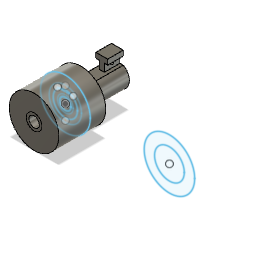
CoilWinder (Autodesk Fusion 360 design; units mm, degrees)
Autodesk Fusion 360 part; units mm, degrees
note: some values were not read from the file. Set by a fixed rule: which sketch regions a step uses.
sketch "Adapter_3mm" plane through (0, 0, 0) normal (0, 0, 1) x (1, 0, 0) in component "Deprecated - Adapter1"
  circle A0 centre (0, 0) radius 1
  circle A1 centre (0, 0) radius 1.5
  circle A2 centre (0, 0) radius 2.3
  circle A3 centre (0, 0) radius 4.7625
  dimension "d1" = 2
  dimension "d2" = 3
  dimension "d3" = 4.6
  dimension "d48" = 9.525
  constraint coincident A0.centre A1.centre
  constraint concentric A0 A1
  constraint concentric A1 A3
  measures "d1" diameter of A0
  measures "d2" diameter of A1
  measures "d3" diameter of A2
  measures "d48" diameter of A3
extrude "Extrude1" add sketch "Adapter_3mm" against normal blind 12 contours A1 | A2 makes body 1 in component "Deprecated - Adapter1"
extrude "Extrude2" add sketch "Adapter_3mm" along normal blind 7 contours A2 bodies 1 in component "Deprecated - Adapter1"
sketch "Face" plane through (0, 0, 0) normal (0, 0, 1) x (1, 0, 0) in component "StepperMount"
  line L0 (0, 0) -> (17.4625, 0) construction
  circle A0 centre (17.4625, 0) radius 1.8
  circle A1 centre (0, 0) radius 4.75
  line L1 (0, 0) -> (0, -15)
  line L2 (0, -15) -> (25, -15)
  line L3 (25, -15) -> (25, 10)
  line L4 (25, 10) -> (0, 10)
  line L5 (0, 10) -> (0, -15)
  line L6 (-25, 10) -> (0, 10)
  line L7 (-25, -15) -> (-25, 10)
  line L8 (0, -15) -> (-25, -15)
  circle A2 centre (-17.4625, 0) radius 1.8
  point P0 (-17.4625, 0)
  dimension "d8" = 17.4625
  dimension "d9" = 3.6
  dimension "d10" = 9.5
  dimension "d11" = 15
  dimension "d12" = 25
  dimension "d13" = 25
  constraint horizontal L0
  constraint coincident L0.start A1.centre
  constraint coincident L0.end A0.centre
  constraint perpendicular L0 L1
  constraint horizontal L2
  constraint vertical L3
  constraint horizontal L4
  constraint vertical L5
  constraint symmetric L0.end L5 P0
  constraint symmetric A0 L5 A2
  constraint symmetric L1.end L5 L2.start
  constraint symmetric L2.end L5 L7.start
  constraint symmetric L3.end L5 L6.start
  constraint symmetric L4.end L5 L6.end
  measures "d8" distance of L0.start L0.end
  measures "d9" diameter of A0
  measures "d10" diameter of A1
  measures "d11" distance of L0.start L1.end
  measures "d12" distance of L1.end L2.end
  measures "d13" distance of L1.end L4.end
ref_plane "WorkPlane1" through (0, -15, 0) normal (0, 1, 0) x (0, 0, 1) in component "StepperMount"
sketch "Base" plane through (0, -15, 0) normal (0, 1, 0) x (1, 0, 0) in component "StepperMount"
  line L0 (0, 0) -> (-25, 0)
  line L1 (0, 0) -> (25, 0)
  line L2 (0, 0) -> (25, 0)
  line L3 (25, 0) -> (25, 18)
  line L4 (25, 18) -> (0, 18)
  line L5 (0, 18) -> (0, 0)
  line L6 (0, 12.9238) -> (19, 12.9238) construction
  circle A0 centre (19, 12.9238) radius 0.95
  line L7 (25, 0) -> (23.4, 0)
  line L8 (23.4, 0) -> (23.4, 18)
  line L9 (23.4, 18) -> (25, 18)
  line L10 (25, 18) -> (25, 0)
  line L11 (-25, 18) -> (0, 18)
  circle A1 centre (-19, 12.9238) radius 0.95
  line L12 (-25, 0) -> (-25, 18)
  line L13 (-23.4, 0) -> (-23.4, 18)
  line L14 (-23.4, 18) -> (-25, 18)
  line L15 (25, 12) -> (30.7822, 8)
  point P0 (-19, 12.9238)
  dimension "d17" = 25
  dimension "d18" = 18
  dimension "d19" = 1.9
  dimension "d20" = 1.6
  dimension "d21" = 18
  constraint horizontal L2
  constraint vertical L3
  constraint horizontal L4
  constraint vertical L5
  constraint coincident L0.start L1.start
  constraint coincident L5 L6.start
  constraint perpendicular L5 L6
  constraint coincident L6.end A0.centre
  constraint horizontal L7
  constraint vertical L8
  constraint horizontal L9
  constraint vertical L10
  constraint symmetric L1.end L5 L0.end
  constraint symmetric L3.end L5 L11.start
  constraint symmetric L4.end L5 L11.end
  constraint symmetric L5 L6.end P0
  constraint symmetric L5 A0 A1
  constraint symmetric L5 L7.end L13.start
  constraint symmetric L5 L8.end L13.end
  constraint symmetric L5 L3.end L11.start
  measures "d17" distance of L0.start L1.end
  measures "d18" distance of L0.start L4.end
  measures "d19" diameter of A0
  measures "d20" distance of L1.end L7.end
  measures "d21" distance of L1.end L3.end
extrude "Extrude1'" add sketch "Face" against normal blind 3 separate body contours A1 L1 L2 L3 L4 L5 | A1 L1 L5 L6 L7 L8 makes body 2 in component "StepperMount"
extrude "Extrude2'" add sketch "Base" against normal blind 3 bodies 2 in component "StepperMount"
extrude "Extrude3" add sketch "Base" along normal blind 25 contours L0 L11 L12 L13 L14 | L1 L2 L3 L4 L7 L8 L9 L10 bodies 2 in component "StepperMount"
fillet "Fillet1" radius 37 2 edges at (24.2, 10, -18) (-24.2, 10, -18) on bodies 2 in component "StepperMount"
sketch "Face (2)" plane through (0, 0, 0) normal (0, 0, 1) x (1, 0, 0) in component "ServoMount"
  line L0 (0, 0) -> (11.75, 0) construction
  line L1 (11.75, 0) -> (17.75, 0)
  line L2 (17.75, 0) -> (17.75, 13.1)
  line L3 (17.75, 13.1) -> (11.75, 13.1)
  line L4 (11.75, 13.1) -> (11.75, 0)
  line L5 (0, 0) -> (0, 7.05) construction
  line L6 (0, 7.05) -> (14, 7.05) construction
  circle A0 centre (14, 7.05) radius 1
  line L7 (-11.75, 13.1) -> (-11.75, 0)
  line L8 (-17.75, 0) -> (-17.75, 13.1)
  line L9 (-17.75, 13.1) -> (-11.75, 13.1)
  line L10 (-11.75, 0) -> (-17.75, 0)
  circle A1 centre (-14, 7.05) radius 1
  point P0 (-14, 7.05)
  dimension "d31" = 11.75
  dimension "d32" = 6
  dimension "d33" = 13.1
  dimension "d36" = 7.05
  dimension "d37" = 14
  dimension "d38" = 2
  constraint coincident L0.start L5.start
  constraint horizontal L0
  constraint horizontal L1
  constraint vertical L2
  constraint horizontal L3
  constraint vertical L4
  constraint vertical L5
  constraint horizontal L6
  constraint coincident L6.end A0.centre
  constraint symmetric L0.end L5 L7.end
  constraint symmetric L1.end L5 L8.start
  constraint symmetric L2.end L5 L8.end
  constraint symmetric L3.end L5 L7.start
  constraint symmetric L5 L6.end P0
  constraint symmetric L5 A0 A1
  measures "d31" distance of L0.start L0.end
  measures "d32" distance of L0.end L1.end
  measures "d33" distance of L0.end L3.end
  measures "d36" distance of L0.start L5.end
  measures "d37" distance of L5.end L6.end
  measures "d38" diameter of A0
sketch "Base (2)" plane through (0, 0, 0) normal (0, 1, 0) x (1, 0, 0) in component "ServoMount"
  line L0 (0, 0) -> (20, 0)
  line L1 (20, 0) -> (20, 15)
  line L2 (20, 15) -> (0, 15)
  line L3 (0, 15) -> (0, 0)
  line L4 (11.75, 0) -> (11.75, 6)
  line L5 (17.75, 0) -> (17.75, 6)
  line L6 (11.75, 6) -> (17.75, 6)
  circle A0 centre (17, 12) radius 0.95
  line L7 (-20, 15) -> (0, 15)
  line L8 (-20, 0) -> (-20, 15)
  line L9 (-11.75, 6) -> (-17.75, 6)
  line L10 (-11.75, 0) -> (-11.75, 6)
  line L11 (-17.75, 0) -> (-17.75, 6)
  line L12 (0, 0) -> (-20, 0)
  circle A1 centre (-17, 12) radius 0.95
  point P0 (-17.75, 0)
  point P1 (17.75, 0)
  point P2 (11.75, 0)
  point P3 (-17.75, 0)
  point P4 (-11.75, 0)
  dimension "d39" = 20
  dimension "d40" = 15
  dimension "d41" = 6
  dimension "d42" = 6
  dimension "d43" = 1.9
  constraint horizontal L0
  constraint vertical L1
  constraint horizontal L2
  constraint vertical L3
  constraint coincident L0.start L3.end
  constraint coincident P2 L4.start
  constraint perpendicular L0 L4
  constraint vertical L5
  constraint coincident P1 L5.start
  constraint symmetric P1 L3 P3
  constraint symmetric L0.start L3 L12.start
  constraint symmetric L0.end L3 L8.start
  constraint symmetric L1.end L3 L7.start
  constraint symmetric L2.end L3 L7.end
  constraint symmetric L3 P2 P4
  constraint symmetric L3 L4.end L9.start
  constraint symmetric L3 P1 P3
  constraint symmetric L3 L5.end L9.end
  constraint symmetric L3 A0 A1
  measures "d39" distance of L0.start L0.end
  measures "d40" distance of L0.start L2.end
  measures "d41" distance of P2 L4.end
  measures "d42" distance of P1 L5.end
  measures "d43" diameter of A0
extrude "Extrude1''" add sketch "Face (2)" against normal blind 6 separate body makes body 3 at (-11.75, 8.7333, -2) makes body 4 at (11.75, 8.7333, -2) in component "ServoMount"
extrude "Extrude2''" add sketch "Base (2)" against normal blind 3 bodies 3 4 in component "ServoMount"
extrude "Extrude3'" add sketch "Adapter_3mm" along normal blind 3 separate body contours A2 | A3 makes body 5 in component "Deprecated - Adapter1"
sketch "Base (3)" plane through (0, 0, 0) normal (0, 0, 1) x (1, 0, 0) in component "Box"
  circle A0 centre (70.0007, 11.7138) radius 1
  line L0 (69.9955, 5.0831) -> (69.9532, 4.8292)
  line L1 (4.0423, 4.8292) -> (4, 5.0831)
  line L2 (6.4219, 57.6265) -> (-6.7489, 57.6265) construction
  line L3 (74.035, 2.5) -> (74.035, 58.8)
  line L4 (4.2962, 57.0924) -> (4.5078, 57.2405)
  circle A1 centre (70.0007, 11.7138) radius 1.5 construction
  line L5 (4.2962, 4.3848) -> (4.127, 4.5964)
  circle A2 centre (17.9705, 6.6261) radius 2.5
  line L6 (4.127, 4.5964) -> (4.0423, 4.8292)
  line L7 (4, 5.0831) -> (4, 56.373)
  circle A3 centre (19.2319, 54.8585) radius 1
  line L8 (76.535, 0) -> (76.535, 61.3)
  line L9 (4, 56.373) -> (4.0423, 56.648)
  line L10 (69.6993, 4.3848) -> (69.4877, 4.2156)
  circle A4 centre (17.9705, 6.6261) radius 1
  line L11 (0, 61.3) -> (0, 0)
  line L12 (69.9955, 55.8652) -> (69.9955, 44.4392)
  line L13 (4.5078, 57.2405) -> (4.7406, 57.3463)
  line L14 (2.5, 58.8) -> (2.5, 2.5)
  line L15 (-0.9239, 7.0886) -> (2.5, 7.0886)
  circle A5 centre (69.9986, 39.6131) radius 1.5 construction
  line L16 (4.7406, 4.1309) -> (4.5078, 4.2156)
  circle A6 centre (69.9986, 39.6131) radius 1
  line L17 (4.0423, 56.648) -> (4.127, 56.8808)
  line L18 (69.9955, 44.4392) -> (72.5346, 41.9001)
  line L19 (1, 60.3) -> (1, 1)
  line L20 (4.9945, 4.0886) -> (4.7406, 4.1309)
  line L21 (69.8686, 4.5964) -> (69.6993, 4.3848)
  line L22 (69.9955, 6.6277) -> (69.9955, 5.0831)
  line L23 (76.535, 61.3) -> (0, 61.3)
  line L24 (1, 1) -> (75.535, 1)
  circle A7 centre (19.2319, 54.8585) radius 2.5
  circle A8 centre (69.9986, 39.6131) radius 2.5
  line L25 (4.9945, 57.3886) -> (68.4721, 57.3886)
  line L26 (2.5, 2.5) -> (74.035, 2.5)
  circle A9 centre (19.2319, 54.8585) radius 1.5 construction
  line L27 (75.535, 60.3) -> (1, 60.3)
  line L28 (74.035, 58.8) -> (2.5, 58.8)
  line L29 (69.001, 4.0886) -> (4.9945, 4.0886)
  line L30 (75.535, 1) -> (75.535, 60.3)
  line L31 (0, 0) -> (76.535, 0)
  line L32 (69.2549, 4.1309) -> (69.001, 4.0886)
  line L33 (72.5346, 9.1668) -> (69.9955, 6.6277)
  line L34 (68.4721, 57.3886) -> (69.9955, 55.8652)
  line L35 (72.5346, 41.9001) -> (72.5346, 9.1668)
  line L36 (4.127, 56.8808) -> (4.2962, 57.0924)
  circle A10 centre (17.9705, 6.6261) radius 1.5 construction
  circle A11 centre (70.0007, 11.7138) radius 2.5
  line L37 (69.4877, 4.2156) -> (69.2549, 4.1309)
  line L38 (69.9532, 4.8292) -> (69.8686, 4.5964)
  line L39 (-0.9239, 4.0886) -> (-0.9239, 7.0886) construction
  line L40 (-3.318, 35.6265) -> (2.5, 35.6265)
  line L41 (-1.8792, 57.6265) -> (-1.8792, 48.6265) construction
  line L42 (-2.7646, 16.5886) -> (2.5, 16.5886)
  line L43 (-2.7646, 4.0886) -> (-2.7646, 16.5886) construction
  line L44 (4.5078, 4.2156) -> (4.2962, 4.3848)
  line L45 (4.7406, 57.3463) -> (4.9945, 57.3886)
  line L46 (-1.8792, 48.6265) -> (2.5, 48.6265)
  line L47 (-3.318, 57.6265) -> (-3.318, 35.6265) construction
  line L48 (7.1962, 4.0886) -> (-5.6422, 4.0886) construction
  dimension "d51" = -2.5
  dimension "d52" = -1
  dimension "d53" = 76.535
  dimension "d54" = 61.3
  dimension "d55" = 3
  dimension "d56" = 9
  dimension "d57" = 22
  dimension "d58" = 12.5
  dimension "d16" = 5
  dimension "d60" = 5
  dimension "d61" = 5
  dimension "d62" = 5
  dimension "d63" = 2
  dimension "d64" = 2
  dimension "d65" = 2
  dimension "d66" = 2
  constraint horizontal L31
  constraint vertical L8
  constraint horizontal L23
  constraint vertical L11
  constraint coincident L11.end L31.start
  constraint coincident L48.start L29
  constraint parallel L29 L48
  constraint coincident L39.start L48
  constraint perpendicular L39 L48
  constraint parallel L2 L25
  constraint vertical L41
  constraint coincident L41.start L2
  constraint perpendicular L2 L41
  constraint vertical L47
  constraint coincident L47.start L2
  constraint vertical L43
  constraint coincident L43.start L48
  constraint perpendicular L43 L48
  constraint coincident L46.end L14
  constraint perpendicular L14 L46
  constraint coincident L40.end L14
  constraint perpendicular L14 L40
  constraint coincident L42.end L14
  constraint perpendicular L14 L42
  constraint coincident L15.end L14
  constraint perpendicular L14 L15
  constraint concentric A2 A10
  constraint concentric A7 A9
  constraint concentric A5 A8
  constraint concentric A1 A11
  constraint concentric A3 A9
  constraint concentric A5 A6
  constraint concentric A0 A1
  constraint concentric A4 A10
  measures "d53" distance of L11.end L8.start
  measures "d54" distance of L11.end L11.start
  measures "d55" distance of L15.start L39.start
  measures "d56" distance of L41.start L41.end
  measures "d57" distance of L47.start L40.start
  measures "d58" distance of L43.start L42.start
  measures "d16" diameter of A2
  measures "d60" diameter of A7
  measures "d61" diameter of A8
  measures "d62" diameter of A11
  measures "d63" diameter of A3
  measures "d64" diameter of A6
  measures "d65" diameter of A0
  measures "d66" diameter of A4
extrude "Extrude1'''" add sketch "Base (3)" against normal blind 1 separate body contours A0 | L0 L1 L4 L5 L6 L7 L9 L10 L12 L13 L16 L17 L18 L20 L21 L22 L25 L29 L32 L33 L34 L35 L36 L37 L38 L44 L45 | L3 L14 L26 L28 | L3 L14 L15 L19 L24 L26 L27 L28 L30 L46 | L14 L15 L19 L42 | L14 L19 L40 L46 | L14 L19 L40 L42 | L8 L11 L15 L19 L23 L24 L27 L30 L31 L46 | L11 L15 L19 L42 | L11 L19 L40 L46 | L11 L19 L40 L42 | A2 | A3 | A4 | A6 | A7 | A8 | A11 makes body 6 in component "Box"
extrude "Extrude2'''" add sketch "Base (3)" along normal blind 4.9 contours L3 L14 L15 L19 L24 L26 L27 L28 L30 L46 | L14 L15 L19 L42 | L14 L19 L40 L46 | L14 L19 L40 L42 | L8 L11 L15 L19 L23 L24 L27 L30 L31 L46 | L11 L15 L19 L42 | L11 L19 L40 L46 | L11 L19 L40 L42 bodies 6 in component "Box"
extrude "Extrude3''" add sketch "Base (3)" along normal blind 8.9 contours L3 L14 L15 L19 L24 L26 L27 L28 L30 L46 | L14 L19 L40 L42 bodies 6 in component "Box"
extrude "Extrude4" add sketch "Base (3)" along normal blind 3.5 contours A2 | A7 | A8 | A11 bodies 6 in component "Box"
sketch "Sides" plane through (0, 0, 4.9) normal (0, 0, 1) x (1, 0, 0) in component "Box"
  line L0 (0, 0) -> (76.535, 0)
  line L1 (76.535, 0) -> (76.535, 61.3)
  line L2 (76.535, 61.3) -> (0, 61.3)
  line L3 (0, 61.3) -> (0, 0)
  line L4 (2.5, 16.5886) -> (1, 16.5886)
  line L5 (1, 16.5886) -> (1, 35.6265)
  line L6 (1, 35.6265) -> (2.5, 35.6265)
  line L7 (2.5, 35.6265) -> (2.5, 48.6265)
  line L8 (2.5, 48.6265) -> (1, 48.6265)
  line L9 (1, 48.6265) -> (1, 60.3)
  line L10 (1, 60.3) -> (75.535, 60.3)
  line L11 (75.535, 60.3) -> (75.535, 1)
  line L12 (75.535, 1) -> (1, 1)
  line L13 (1, 1) -> (1, 7.0886)
  line L14 (1, 7.0886) -> (2.5, 7.0886)
  line L15 (2.5, 7.0886) -> (2.5, 16.5886)
  line L16 (2.5, 7.0886) -> (1, 7.0886)
  line L17 (1, 7.0886) -> (1, 1)
  line L18 (1, 1) -> (75.535, 1)
  line L19 (75.535, 1) -> (75.535, 60.3)
  line L20 (75.535, 60.3) -> (1, 60.3)
  line L21 (1, 60.3) -> (1, 48.6265)
  line L22 (1, 48.6265) -> (2.5, 48.6265)
  line L23 (2.5, 35.6265) -> (2.5, 48.6265)
  line L24 (2.5, 35.6265) -> (1, 35.6265)
  line L25 (1, 35.6265) -> (1, 16.5886)
  line L26 (1, 16.5886) -> (2.5, 16.5886)
  line L27 (2.5, 7.0886) -> (2.5, 16.5886)
  line L28 (2.5, 2.5) -> (2.5, 7.0886)
  line L29 (74.035, 2.5) -> (2.5, 2.5)
  line L30 (74.035, 58.8) -> (74.035, 2.5)
  line L31 (2.5, 58.8) -> (74.035, 58.8)
  line L32 (2.5, 48.6265) -> (2.5, 58.8)
  line L33 (2.5, 16.5886) -> (2.5, 35.6265)
  line L34 (76.535, 0) -> (76.535, 61.3)
  line L35 (76.535, 61.3) -> (0, 61.3)
  line L36 (0, 61.3) -> (0, 0)
  line L37 (0, 0) -> (76.535, 0)
  line L38 (-2.7646, 16.5886) -> (2.5, 16.5886)
  line L39 (-0.9239, 7.0886) -> (2.5, 7.0886)
  line L40 (-1.8792, 48.6265) -> (2.5, 48.6265)
  line L41 (-3.318, 35.6265) -> (2.5, 35.6265)
  line L42 (74.535, 59.3) -> (2, 59.3)
  line L43 (2, 59.3) -> (2, 2)
  line L44 (2, 2) -> (74.535, 2)
  line L45 (74.535, 2) -> (74.535, 59.3)
  dimension "d77" = -2
extrude "Extrude5" add sketch "Sides" along normal blind 50 separate body contours L0 L1 L2 L3 L9 L10 L11 L12 L13 L17 L18 L19 L20 L21 L34 L35 L36 L37 L39 L40 | L3 L4 L14 L16 L26 L36 L38 L39 L43 | L3 L5 L25 L36 L38 L41 | L8 L9 L10 L11 L12 L13 L14 L16 L17 L18 L19 L20 L21 L22 L39 L40 L42 L43 L44 L45 | L3 L6 L8 L22 L24 L36 L40 L41 L43 | L4 L5 L6 L24 L25 L26 L38 L41 L43 makes body 7 in component "Box"
extrude "Extrude6" cut sketch "Sides" along normal blind 12 contours L3 L4 L14 L16 L26 L36 L38 L39 L43 | L3 L6 L8 L22 L24 L36 L40 L41 L43 bodies 7 in component "Box"
combine "Combine1" operation cut target body 7 tool bodies 6 keep tools in component "Box"
sketch "DisplayFace" plane through (0, 0, 0) normal (0, -1, 0) x (1, 0, 0) in component "Box"
  line L0 (0, 4.9) -> (76.535, 4.9)
  line L1 (76.535, 4.9) -> (76.535, 54.9)
  line L2 (76.535, 54.9) -> (0, 54.9)
  line L3 (0, 54.9) -> (0, 4.9)
  line L4 (0, 4.9) -> (30, 4.9) construction
  line L5 (30, 4.9) -> (30, 30.9) construction
  line L6 (30, 30.9) -> (58, 30.9)
  line L7 (58, 30.9) -> (58, 43.9)
  line L8 (58, 43.9) -> (30, 43.9)
  line L9 (30, 43.9) -> (30, 30.9)
  point P0 (0, 4.9)
  dimension "d80" = 30
  dimension "d81" = 26
  dimension "d82" = 28
  dimension "d83" = 13
  constraint horizontal L4
  constraint coincident P0 L0.start
  constraint vertical L5
  constraint horizontal L6
  constraint vertical L7
  constraint horizontal L8
  constraint vertical L9
  measures "d80" distance of P0 L4.end
  measures "d81" distance of L4.end L5.end
  measures "d82" distance of L5.end L6.end
  measures "d83" distance of L5.end L8.end
sketch "ButtonFace" plane through (76.535, 0, 0) normal (1, 0, 0) x (0, 0, -1) in component "Box"
  line L0 (-4.9, 0) -> (-4.9, 61.3)
  line L1 (-4.9, 61.3) -> (-54.9, 61.3)
  line L2 (-54.9, 61.3) -> (-54.9, 0)
  line L3 (-54.9, 0) -> (-4.9, 0)
  line L4 (-4.9, 43.65) -> (-30.9, 43.65) construction
  circle A0 centre (-30.9, 43.65) radius 3.5
  line L5 (-24.9, 49.65) -> (-36.9, 49.65) construction
  line L6 (-36.9, 49.65) -> (-36.9, 37.65) construction
  line L7 (-36.9, 37.65) -> (-24.9, 37.65) construction
  line L8 (-24.9, 37.65) -> (-24.9, 49.65) construction
  line L9 (-24.9, 49.65) -> (-36.9, 37.65) construction
  line L10 (-36.9, 49.65) -> (-24.9, 37.65) construction
  line L11 (-29.4, 50.15) -> (-32.4, 50.15)
  line L12 (-32.4, 50.15) -> (-32.4, 49.15)
  line L13 (-32.4, 49.15) -> (-29.4, 49.15)
  line L14 (-29.4, 49.15) -> (-29.4, 50.15)
  line L15 (-29.4, 50.15) -> (-32.4, 49.15) construction
  line L16 (-32.4, 50.15) -> (-29.4, 49.15) construction
  point P0 (-30.9, 43.65)
  point P1 (-30.9, 49.65)
  dimension "d84" = 26
  dimension "d85" = 7
  dimension "d232" = 12
  dimension "d233" = 12
  dimension "d234" = 3
  dimension "d235" = 1
  constraint horizontal L4
  constraint coincident P0 L4.end
  constraint horizontal L5
  constraint perpendicular L5 L6
  constraint parallel L5 L7
  constraint parallel L6 L8
  constraint coincident L9 P0
  constraint coincident L10 P0
  constraint horizontal L11
  constraint perpendicular L11 L12
  constraint parallel L11 L13
  constraint parallel L12 L14
  constraint coincident L15 P1
  constraint coincident L16 P1
  constraint midpoint L5 P1
  measures "d84" distance of L4.start P0
  measures "d85" diameter of A0
  measures "d232" distance of L6.end L7.end
  measures "d233" distance of L5.end L6.end
  measures "d234" distance of L12.end L13.end
  measures "d235" distance of L11.end L12.end
extrude "Extrude7" cut sketch "DisplayFace" against normal blind 3 contours L6 L7 L8 L9 bodies 7 in component "Box"
extrude "Extrude8" cut sketch "ButtonFace" against normal blind 3 contours A0 | L11 L12 L13 L14 bodies 7 in component "Box"
extrude "Extrude10" add sketch "ButtonFace" against normal blind 1 contours L11 L12 L13 L14 bodies 7 in component "Box"
sketch "Flange" plane through (0, 0, 54.9) normal (0, 0, 1) x (1, 0, 0) in component "Box"
  line L0 (74.535, 59.3) -> (74.535, 2)
  line L1 (74.535, 2) -> (2, 2)
  line L2 (2, 2) -> (2, 59.3)
  line L3 (2, 59.3) -> (74.535, 59.3)
  line L4 (0, 0) -> (76.535, 0)
  line L5 (76.535, 0) -> (76.535, 61.3)
  line L6 (76.535, 61.3) -> (0, 61.3)
  line L7 (0, 61.3) -> (0, 0)
  line L8 (2, 2) -> (2, 59.3)
  line L9 (2, 59.3) -> (74.535, 59.3)
  line L10 (74.535, 59.3) -> (74.535, 2)
  line L11 (74.535, 2) -> (2, 2)
  line L12 (0, 61.3) -> (0, 0)
  line L13 (0, 0) -> (76.535, 0)
  line L14 (76.535, 0) -> (76.535, 61.3)
  line L15 (76.535, 61.3) -> (0, 61.3)
  line L16 (-6, -6) -> (82.535, -6)
  line L17 (82.535, -6) -> (82.535, 67.3)
  line L18 (82.535, 67.3) -> (-6, 67.3)
  line L19 (-6, 67.3) -> (-6, -6)
  line L20 (76.535, 61.3) -> (82.535, 67.3) construction
  circle A0 centre (79.535, 64.3) radius 0.75
  line L21 (0, 61.3) -> (-6, 67.3) construction
  line L22 (-6, -6) -> (0, 0) construction
  line L23 (82.535, -6) -> (76.535, 0) construction
  circle A1 centre (-3, 64.3) radius 0.75
  circle A2 centre (-3, -3) radius 0.75
  circle A3 centre (79.535, -3) radius 0.75
  dimension "d90" = 6
  dimension "d91" = 1.5
  dimension "d92" = 1.5
  dimension "d93" = 1.5
  dimension "d94" = 1.5
  constraint coincident L5.end L6.start
  constraint midpoint L20 A0.centre
  constraint coincident L6.end L7.start
  constraint coincident L4.start L7.end
  constraint coincident L4.end L5.start
  constraint midpoint L21 A1.centre
  constraint midpoint L22 A2.centre
  constraint midpoint L23 A3.centre
  measures "d91" diameter of A0
  measures "d92" diameter of A1
  measures "d93" diameter of A2
  measures "d94" diameter of A3
extrude "Extrude9" add sketch "Flange" against normal blind 2 contours L16 L17 L18 L19 bodies 7 in component "Box"
sketch "Left" plane through (0, 0, 0) normal (0, 0, 1) x (1, 0, 0) in component "OLEDHolder"
  line L0 (0, 0) -> (5, 0)
  line L1 (5, 0) -> (5, 2.4)
  line L2 (5, 2.4) -> (17.3, 2.4)
  line L3 (17.3, 2.4) -> (17.3, 1.9)
  line L4 (17.3, 1.9) -> (18.8, 1.9)
  line L5 (18.8, 1.9) -> (18.8, 3.5)
  line L6 (18.8, 3.5) -> (0, 3.5)
  line L7 (0, 3.5) -> (0, 0)
  line L8 (5, 2.4) -> (5, 3.5)
  dimension "d98" = 5
  dimension "d99" = 2.4
  dimension "d100" = 12.3
  dimension "d101" = 0.5
  dimension "d109" = 1.5
  constraint horizontal L0
  constraint coincident L0.start L7.end
  constraint vertical L1
  constraint horizontal L2
  constraint vertical L3
  constraint perpendicular L3 L4
  constraint perpendicular L4 L5
  constraint perpendicular L3 L6
  constraint perpendicular L0 L7
  constraint coincident L6 L8.end
  constraint perpendicular L6 L8
  measures "d98" distance of L0.start L0.end
  measures "d99" distance of L0.end L1.end
  measures "d100" distance of L1.end L2.end
  measures "d101" distance of L2.end L3.end
  measures "d109" distance of L3.end L4.end
ref_plane "WorkPlane1" through (0, 0, -32) normal (0, 0, 1) x (1, 0, 0) in component "OLEDHolder"
sketch "Right" plane through (0, 0, -32) normal (0, 0, 1) x (1, 0, 0) in component "OLEDHolder"
  line L0 (0, 3.5) -> (0, 0)
  line L1 (18.8, 3.5) -> (0, 3.5)
  line L2 (5, 2.4) -> (17.3, 2.4)
  line L3 (5, 0) -> (5, 2.4)
  line L4 (0, 0) -> (5, 0)
  line L5 (18.8, 1.9) -> (18.8, 3.5)
  line L6 (17.3, 1.9) -> (18.8, 1.9)
  line L7 (17.3, 2.4) -> (17.3, 1.9)
extrude "Extrude1''''" add sketch "Left" against normal blind 4 separate body makes body 8 in component "OLEDHolder"
extrude "Extrude2''''" add sketch "Left" against normal blind 32 contours L0 L1 L6 L7 L8 bodies 8 in component "OLEDHolder"
extrude "Extrude3'''" add sketch "Right" against normal blind 4 bodies 8 in component "OLEDHolder"
sketch "TopView" plane through (0, 0, 0) normal (0, 1, 0) x (1, 0, 0) in component "SpoolHolder"
  line L0 (0, 0) -> (10, 0)
  line L1 (10, 0) -> (10, 10)
  line L2 (10, 10) -> (0, 10)
  line L3 (0, 10) -> (0, 0)
  line L4 (10, 5) -> (17, 5) construction
  line L5 (17, 5) -> (17, 20) construction
  line L6 (17, 20) -> (23, 20)
  line L7 (23, 20) -> (23, 24)
  line L8 (23, 24) -> (17, 24)
  line L9 (17, 24) -> (17, 20)
  line L10 (11, 24) -> (17, 24)
  line L11 (11, 20) -> (11, 24)
  line L12 (17, 20) -> (11, 20)
  line L13 (0, 0) -> (23, 0)
  line L14 (23, 0) -> (23, 24)
  line L15 (23, 24) -> (0, 24)
  line L16 (0, 24) -> (0, 0)
  circle A0 centre (3, 21) radius 0.95
  circle A1 centre (20, 3) radius 0.95
  dimension "d110" = 10
  dimension "d111" = 10
  dimension "d112" = 7
  dimension "d113" = 15
  dimension "d114" = 6
  dimension "d115" = 4
  dimension "d116" = 23
  dimension "d117" = 24
  dimension "d118" = 1.9
  dimension "d119" = 1.9
  constraint horizontal L0
  constraint vertical L1
  constraint horizontal L2
  constraint vertical L3
  constraint horizontal L4
  constraint midpoint L1 L4.start
  constraint vertical L5
  constraint horizontal L6
  constraint vertical L7
  constraint horizontal L8
  constraint vertical L9
  constraint symmetric L5.end L9 L6.start
  constraint symmetric L6.end L9 L11.start
  constraint symmetric L7.end L9 L10.start
  constraint symmetric L8.end L9 L10.end
  constraint horizontal L13
  constraint vertical L14
  constraint horizontal L15
  constraint vertical L16
  constraint coincident L0.start L3.end
  measures "d110" distance of L0.start L0.end
  measures "d111" distance of L0.start L2.end
  measures "d112" distance of L4.start L4.end
  measures "d113" distance of L4.end L5.end
  measures "d114" distance of L5.end L6.end
  measures "d115" distance of L5.end L8.end
  measures "d116" distance of L0.start L13.end
  measures "d117" distance of L0.start L15.end
  measures "d118" diameter of A0
  measures "d119" diameter of A1
extrude "Extrude1'''''" add sketch "TopView" against normal blind 1 separate body makes body 9 in component "SpoolHolder"
extrude "Extrude2'''''" add sketch "TopView" along normal blind 19 contours L0 L1 L2 L3 L13 L16 bodies 9 in component "SpoolHolder"
extrude "Extrude3''''" add sketch "TopView" along normal blind 20 contours L6 L7 L8 L9 L14 L15 | L9 L10 L11 L12 L15 bodies 9 in component "SpoolHolder"
sketch "SideView" plane through (0, 0, 0) normal (1, 0, 0) x (0, 0, -1) in component "SpoolHolder"
  line L0 (0, 0) -> (5, 0) construction
  line L1 (5, 0) -> (5, 13) construction
  circle A0 centre (5, 13) radius 2.8
  circle A1 centre (5, 13) radius 10 construction
  dimension "d126" = 5
  dimension "d127" = 13
  dimension "d128" = 5.6
  dimension "d129" = 20
  constraint horizontal L0
  constraint coincident L0.start origin
  constraint vertical L1
  constraint coincident L1.end A0.centre
  constraint concentric A0 A1
  measures "d126" distance of L0.start L0.end
  measures "d127" distance of L0.end L1.end
  measures "d128" diameter of A0
  measures "d129" diameter of A1
extrude "Extrude4'" cut sketch "SideView" along normal blind 21 bodies 9 in component "SpoolHolder"
ref_plane "WorkPlane1" through (25, 0, 0) normal (1, 0, 0) x (0, 1, 0) in component "SpoolHolder"
sketch "Washer" plane through (25, 0, 0) normal (1, 0, 0) x (0, 0, -1) in component "SpoolHolder"
  circle A0 centre (5, 13) radius 2.825
  circle A1 centre (5, 13) radius 5.825
  point P0 (5, 13)
  dimension "d133" = 5.65
  dimension "d134" = 3
  constraint coincident P0 A0.centre
  measures "d133" diameter of A0
extrude "Extrude5'" add sketch "Washer" along normal blind 3 separate body makes body 10 in component "SpoolHolder"
sketch "AlumTube" plane through (0, 0, 0) normal (1, 0, 0) x (0, 0, -1) in component "SpoolHolder"
  circle A0 centre (5, 13) radius 2.8
  circle A1 centre (5, 13) radius 2.3
  point P0 (5, 13)
  dimension "d137" = 5.6
  dimension "d138" = -0.5
  constraint coincident P0 A0.centre
  measures "d137" diameter of A0
extrude "Extrude6'" add sketch "AlumTube" along normal blind 28 separate body makes body 11 in component "SpoolHolder"
ref_plane "WorkPlane2" through (12, 9.5, -5) normal (1, 0, 0) x (0, 0, -1) in component "SpoolHolder"
sketch "Sketch6" plane through (12, 9.5, -5) normal (1, 0, 0) x (0, 0, -1) in component "SpoolHolder"
  circle A0 centre (0, 3.5) radius 2.8
  circle A1 centre (0, 3.5) radius 4.8
  dimension "d142" = 2
extrude "Extrude7'" add sketch "Sketch6" along normal blind 11 separate body makes body 12 in component "SpoolHolder"
sketch "Spacers" plane through (0, 0, 0) normal (0, 0, 1) x (1, 0, 0) in component "Spacers"
  circle A0 centre (4, 5) radius 2
  line L0 (0, 5) -> (8, 5)
  line L1 (8, 5) -> (8, 10)
  line L2 (8, 10) -> (0, 10)
  line L3 (0, 10) -> (0, 5)
  dimension "d145" = 4
  dimension "d146" = 8
  dimension "d147" = 5
  constraint horizontal L0
  constraint vertical L1
  constraint horizontal L2
  constraint vertical L3
  measures "d145" diameter of A0
  measures "d146" distance of L0.start L0.end
  measures "d147" distance of L0.start L2.end
extrude "Extrude1''''''" add sketch "Spacers" along normal blind 3 separate body contours A0 L0 L1 L2 L3 makes body 13 in component "Spacers"
sketch "SpoolAdapter" plane through (0, 0, 0) normal (0, 0, 1) x (1, 0, 0) in component "Deprecated - Adapter1"
  circle A0 centre (0, 0) radius 1.5
  circle A1 centre (0, 0) radius 3.1
  circle A2 centre (0, 0) radius 0.5
  dimension "d150" = 3
  dimension "d151" = 6.2
  dimension "d156" = 1
  constraint coincident A0.centre A1.centre
  constraint concentric A0 A1
  constraint concentric A0 A2
  measures "d150" diameter of A0
  measures "d151" diameter of A1
  measures "d156" diameter of A2
extrude "Extrude4''" add sketch "SpoolAdapter" along normal blind 10 separate body contours A0 | A1 makes body 14 in component "Deprecated - Adapter1"
extrude "Extrude5''" add sketch "SpoolAdapter" against normal blind 6 contours A0 bodies 14 in component "Deprecated - Adapter1"
chamfer "Chamfer1" distance 0.4 angle 45 1 edges at (-1.3985, 0.5424, -6) on bodies 14 in component "Deprecated - Adapter1"
chamfer "Chamfer2" distance 0.2 angle 45 2 edges at (-2.8902, -1.121, 0) (-2.8902, -1.121, 10) on bodies 14 in component "Deprecated - Adapter1"
sketch "Profile" plane through (0, 0, 0) normal (0, 0, 1) x (1, 0, 0) in component "Deprecated - Adapter2"
  circle A0 centre (0, 0) radius 4.7625
  circle A1 centre (0, 0) radius 1.5
  circle A2 centre (0, 0) radius 2.3
  circle A3 centre (0, 0) radius 1
  line L0 (-1.5, 1) -> (1.4, 1)
  circle A4 centre (-3, 0) radius 0.85
  line L1 (0, 3) -> (0, -2.8) construction
  circle A5 centre (3, 0) radius 0.85
  dimension "d163" = 2
  dimension "d164" = 3
  dimension "d165" = 4.6
  dimension "d166" = 9.525
  dimension "d183" = 1.7
  constraint coincident A0.centre A1.centre
  constraint concentric A1 A3
  constraint concentric A0 A1
  constraint horizontal L0
  constraint vertical L1
  constraint symmetric A4 L1 A5
  measures "d163" diameter of A3
  measures "d164" diameter of A1
  measures "d165" diameter of A2
  measures "d166" diameter of A0
  measures "d183" diameter of A4
extrude "Extrude1'''''''" add sketch "Profile" against normal blind 13 separate body contours A1 L0 | A1 L0 | A2 A5 | A2 A4 A5 | A2 A4 picked at (2.2493, -0.0679) picked at (-2.2471, 0) makes body 15 in component "Deprecated - Adapter2"
extrude "Extrude2''''''" add sketch "Profile" against normal blind 3 contours A0 | A2 A5 | A2 A4 picked at (3.3303, 0.0412) picked at (-2.813, -0.0212) bodies 15 in component "Deprecated - Adapter2"
extrude "Extrude3'''''" cut sketch "Profile" against normal blind 3 contours A1 L0 picked at (-1.1441, -0.6793) bodies 15 in component "Deprecated - Adapter2"
extrude "Extrude8'" cut sketch "Profile" against normal blind 1.1 contours A2 A5 | A2 A5 | A2 A4 | A2 A4 bodies 15 in component "Deprecated - Adapter2"
extrude "Extrude4'''" add sketch "Profile" along normal blind 7 separate body contours A0 | A2 A5 | A2 A5 | A2 A4 A5 | A2 A4 | A2 A4 makes body 16 in component "Deprecated - Adapter2"
extrude "Extrude6''" add sketch "Profile" along normal blind 3 and the other way blind 2 contours A3 | A1 L0 picked at (-1.1441, -0.6793) bodies 16 in component "Deprecated - Adapter2"
extrude "Extrude7''" add sketch "Profile" along normal blind 2 contours A1 L0 picked at (-0.0699, 1.3284) bodies 16 in component "Deprecated - Adapter2"
extrude "Extrude9'" cut sketch "Profile" along normal blind 1.1 contours A2 A5 | A2 A5 | A2 A4 | A2 A4 bodies 16 in component "Deprecated - Adapter2"
sketch "Profile (2)" plane through (0, 0, 0) normal (0, 0, 1) x (1, 0, 0) in component "SpindleAdapters"
  circle A0 centre (0, 0) radius 4.7625
  circle A1 centre (0, 0) radius 1.5
  circle A2 centre (0, 0) radius 1
  line L0 (0, 3) -> (0, -2.8) construction
  circle A3 centre (0, 0) radius 2.3
  line L1 (-1.5, 2) -> (1.5, 2)
  circle A4 centre (0, 0) radius 1.05
  circle A5 centre (20, 0) radius 2.85
  circle A6 centre (20, 0) radius 4.85
  circle A7 centre (0, 0) radius 1.16
  circle A8 centre (0, 0) radius 2.35
  line L2 (-1.5, 2.05) -> (1.5, 2.05)
  circle A9 centre (0, 0) radius 3.1
  dimension "d188" = 2
  dimension "d189" = 3
  dimension "d190" = 4.6
  dimension "d191" = 9.525
  dimension "d197" = 2.1
  dimension "d206" = 5.7
  dimension "d207" = 2
  dimension "d214" = 2.32
  dimension "d215" = 0.05
  dimension "d216" = -0.05
  dimension "d238" = 6.2
  constraint coincident A0.centre A1.centre
  constraint concentric A1 A2
  constraint concentric A0 A1
  constraint vertical L0
  constraint horizontal L1
  constraint concentric A0 A4
  constraint concentric A2 A7
  constraint concentric A1 A9
  measures "d188" diameter of A2
  measures "d189" diameter of A1
  measures "d190" diameter of A3
  measures "d191" diameter of A0
  measures "d197" diameter of A4
  measures "d206" diameter of A5
  measures "d214" diameter of A7
  measures "d238" diameter of A9
extrude "Extrude1''''''''" add sketch "Profile (2)" against normal blind 10 separate body contours A1 | A3 L1 | A4 | A7 makes body 17 in component "SpindleAdapters"
sketch "WireCatch" plane through (0, 0, -10) normal (0, 0, -1) x (-1, 0, 0) in component "SpindleAdapters"
  circle A0 centre (0, 0) radius 1
  arc A1 (-1.1358, 2) -> (1.1358, 2) centre (0, 0) ccw
  line L0 (1.1358, 2) -> (-1.1358, 2)
  line L1 (-1.1358, 4.5) -> (1.1358, 4.5)
  line L2 (1.1358, 4.5) -> (1.1358, 2)
  line L3 (1.1358, 2) -> (-1.1358, 2)
  line L4 (-1.1358, 2) -> (-1.1358, 4.5)
  line L5 (0.5, 5) -> (0.5, 2)
  line L6 (-0.5, 5) -> (-0.5, 2)
  line L7 (1.5, 3.5) -> (-1.5, 3.5)
  constraint horizontal L1
  constraint vertical L2
  constraint horizontal L3
  constraint vertical L4
  constraint coincident A1.start L0.end
  constraint coincident A1.end L0.start
  constraint coincident L3 L5.end
  constraint perpendicular L3 L5
  constraint coincident L0 L6.end
  constraint perpendicular L0 L6
  constraint perpendicular L4 L7
extrude "Extrude4''''" add sketch "WireCatch" against normal blind 3 contours L0 L3 L5 L6 L7 | L1 L4 L6 L7 | L1 L2 L5 L7 | L1 L5 L6 L7 bodies 17 in component "SpindleAdapters"
hole "Hole1" at (0.5, 2.8071, -8.5) direction (-1, 0, 0) diameter 0.6 depth 1 tip angle 118 bodies 17 in component "SpindleAdapters"
extrude "Extrude5'''" add sketch "Profile (2)" along normal blind 3 separate body contours A6 makes body 18 in component "SpindleAdapters"
extrude "Extrude2'''''''" add sketch "Profile (2)" against normal blind 3 separate body contours A0 | A3 L2 | A3 A8 L2 | A9 makes body 19 in component "SpindleAdapters"
extrude "Extrude3''''''" add sketch "Profile (2)" along normal blind 6 contours A0 | A1 | A3 L1 | A3 L1 A8 | A3 L1 L2 | A3 L1 A8 L2 | A3 L1 A8 L2 | A3 L2 | A3 A8 L2 | A4 | A7 | A9 bodies 19 in component "SpindleAdapters"
extrude "Extrude6'''" add sketch "Profile (2)" against normal blind 3 separate body contours A0 | A3 L2 | A3 A8 L2 | A9 makes body 20 in component "SpindleAdapters"
extrude "Extrude7'''" add sketch "Profile (2)" along normal blind 6 contours A0 | A3 L1 | A3 L1 A8 | A3 L1 L2 | A3 L1 A8 L2 | A3 L1 A8 L2 | A3 L2 | A3 A8 L2 | A9 bodies 20 in component "SpindleAdapters"
extrude "Extrude8''" add sketch "Profile (2)" against normal blind 3 separate body contours A0 | A3 L2 | A3 A8 L2 | A9 makes body 21 in component "SpindleAdapters"
extrude "Extrude9''" add sketch "Profile (2)" along normal blind 6 contours A0 | A1 | A3 L1 | A3 L1 A8 | A3 L1 L2 | A3 L1 A8 L2 | A3 L1 A8 L2 | A3 L2 | A3 A8 L2 | A9 bodies 21 in component "SpindleAdapters"
sketch "TubeCutter" plane through (0, 0, 0) normal (0, 0, 1) x (1, 0, 0) in component "SpindleAdapters"
  circle A0 centre (12.9317, -0.04) radius 2.5
  circle A1 centre (12.9317, -0.04) radius 5.5
  circle A2 centre (0, 0) radius 5.8
  circle A3 centre (0, 0) radius 2.8
  circle A4 centre (26, 0) radius 5.55
  circle A5 centre (26, 0) radius 2.55
  dimension "d221" = 3
  dimension "d222" = 5
  dimension "d223" = 3
  dimension "d224" = 5.6
  dimension "d225" = 3
  dimension "d226" = 5.1
  measures "d222" diameter of A0
  measures "d224" diameter of A3
  measures "d226" diameter of A5
extrude "Extrude10'" add sketch "TubeCutter" along normal blind 3 separate body makes body 22 at (31.5431, -0.2766, 2) makes body 23 at (18.4249, -0.3142, 2) makes body 24 at (5.7928, -0.2891, 2) in component "SpindleAdapters"
extrude "Extrude11" add sketch "Profile (2)" against normal blind 3 separate body contours A0 | A3 L2 | A3 A8 L2 | A9 makes body 25 in component "SpindleAdapters"
extrude "Extrude12" add sketch "Profile (2)" along normal blind 16 contours A1 | A2 | A3 L1 | A3 L1 A8 | A3 L1 L2 | A3 L1 A8 L2 | A3 L1 A8 L2 | A3 L2 | A3 A8 L2 | A4 | A7 | A9 bodies 25 in component "SpindleAdapters"
extrude "Extrude13" add sketch "Profile (2)" along normal blind 3 contours A0 bodies 25 in component "SpindleAdapters"
sketch "Spool" plane through (0, 0, 0) normal (0, 0, 1) x (1, 0, 0) in component "BigSpoolHolder"
  circle A0 centre (0, 0) radius 1.5
  circle A1 centre (0, 0) radius 9.8
  circle A2 centre (0, 0) radius 22 construction
  dimension "d245" = 3
  dimension "d246" = 19.6
  dimension "d250" = 44
  constraint coincident A0.centre A1.centre
  constraint concentric A1 A2
  measures "d245" diameter of A0
  measures "d246" diameter of A1
  measures "d250" diameter of A2
sketch "Holder" plane through (0, 0, 0) normal (0, 0, 1) x (1, 0, 0) in component "BigSpoolHolder"
  circle A0 centre (0, 0) radius 3.05
  line L0 (-5, 5) -> (5, 5)
  line L1 (5, 5) -> (5, -23)
  line L2 (5, -23) -> (-5, -23)
  line L3 (-5, -23) -> (-5, 5)
  line L4 (-5, -23) -> (5, -23)
  line L5 (5, -23) -> (5, -26)
  line L6 (5, -26) -> (-5, -26)
  line L7 (-5, -26) -> (-5, -23)
  circle A1 centre (0, 0) radius 2
  dimension "d247" = 6.1
  dimension "d248" = 10
  dimension "d249" = 28
  dimension "d251" = 10
  dimension "d252" = 3
  dimension "d261" = 4
  constraint coincident A0.centre A1.centre
  constraint horizontal L0
  constraint vertical L1
  constraint horizontal L2
  constraint vertical L3
  constraint horizontal L4
  constraint vertical L5
  constraint horizontal L6
  constraint vertical L7
  measures "d247" diameter of A0
  measures "d248" distance of L0.start L0.end
  measures "d249" distance of L0.start L2.end
  measures "d251" distance of L2.end L1.end
  measures "d252" distance of L2.end L6.end
  measures "d261" diameter of A1
extrude "Extrude1'''''''''" add sketch "Spool" along normal blind 10 separate body makes body 26 in component "BigSpoolHolder"
extrude "Extrude2''''''''" add sketch "Holder" along normal blind 2.6 separate body contours L0 L1 L2 L3 L4 | L2 L4 L5 L6 L7 makes body 27 in component "BigSpoolHolder"
extrude "Extrude3'''''''" add sketch "Holder" along normal blind 18 contours L2 L4 L5 L6 L7 bodies 27 in component "BigSpoolHolder"
extrude "Extrude4'''''" add sketch "Holder" against normal blind 0.4 contours A0 | L0 L1 L2 L3 L4 | L2 L4 L5 L6 L7 bodies 27 in component "BigSpoolHolder"
sketch "Holes" plane through (0, 0, 0) normal (0, 1, 0) x (1, 0, 0) in component "BigSpoolHolder"
  line L0 (0, 0) -> (0, -20) construction
  circle A0 centre (0, -14) radius 1
  circle A1 centre (0, -8) radius 1
  point P0 (0, -8)
  point P1 (0, -14)
  constraint coincident L0.start origin
  constraint vertical L0
  constraint coincident L0 P0
  constraint coincident L0 P1
  constraint coincident P1 A0.centre
  constraint coincident P0 A1.centre
extrude "Extrude5''''" cut sketch "Holes" against normal blind 29 bodies 27 in component "BigSpoolHolder"
fillet "Fillet3" radius 2 1 edges at (0, -23, 2.6) on bodies 27 in component "BigSpoolHolder"
fillet "Fillet4" radius 2 2 edges at (-5, -24.5, 18) (5, -24.5, 18) on bodies 27 in component "BigSpoolHolder"
fillet "Fillet5" radius 3 2 edges at (-5, 5, 1.1) (5, 5, 1.1) on bodies 27 in component "BigSpoolHolder"
component "ServoMount" placed x (1, 0, 0) y (0, 1, 0) z (0, 0, 1) at (0, 0, 0)
component "Box" placed x (1, 0, 0) y (0, 1, 0) z (0, 0, 1) at (0, 0, 0)
component "OLEDHolder" placed x (1, 0, 0) y (0, 1, 0) z (0, 0, 1) at (0, 0, 0)
component "SpoolHolder" placed x (1, 0, 0) y (0, 1, 0) z (0, 0, 1) at (0, 0, 0)
component "Spacers" placed x (1, 0, 0) y (0, 1, 0) z (0, 0, 1) at (0, 0, 0)
component "Deprecated - Adapter1" placed x (1, 0, 0) y (0, 1, 0) z (0, 0, 1) at (0, 0, 0)
component "Deprecated - Adapter2" placed x (1, 0, 0) y (0, 1, 0) z (0, 0, 1) at (0, 0, 0)
component "SpindleAdapters" placed x (1, 0, 0) y (0, 1, 0) z (0, 0, 1) at (0, 0, 0)
component "BigSpoolHolder" placed x (1, 0, 0) y (0, 1, 0) z (0, 0, 1) at (0, 0, 0)
component "StepperMount" placed x (1, 0, 0) y (0, 1, 0) z (0, 0, 1) at (0, 0, 0) in component "ServoMount"
hidden bodies 6 16 18 21 22 23 24 25
named bodies: "Adapter_3mm", "StepperMount", "ServoMount", "Washer", "Base", "Sides", "OLEDHolder", "SpoolHolder", "AlumTube", "Bobbin", "3mm", "SpoolAdapter", "Adapter", "Spindle", "2mm", "TubeCutter", "2.4mm", "TubeCutter5_6", "TubeCutter5", "TubeCutter5_1", "BobbinHolder", "Spool", "Holder"
